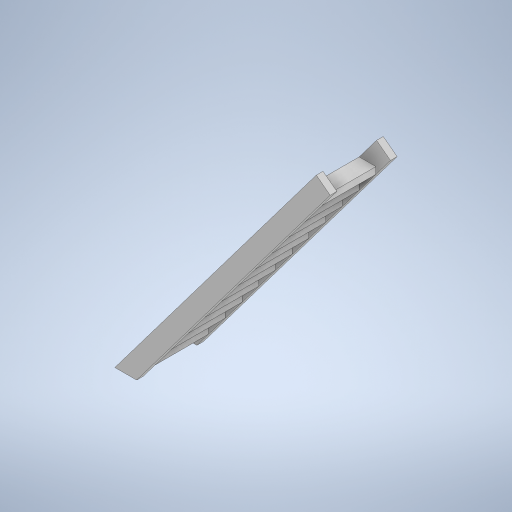
# Autodesk Inventor part: Maitri_Ladder
Saved by Autodesk Inventor 2023 (Build 270158000, 158)
## iProperties
Created: 2023-09-22
Part Number: Maitri_Ladder
Material: Generic
Document SubType Name: Modeling
Designer: maitr
Density: 1 g/cm^3
Appearance: Default
Author: maitr
Autodesk Inventor part; units mm, degrees
ref_plane "YZ Plane" through (0, 0, 0) normal (1, 0, 0) x (0, 1, 0)
ref_plane "XZ Plane" through (0, 0, 0) normal (0, 1, 0) x (-1, 0, 0)
sketch "Sketch1" plane through (0, 0, 0) normal (0, 0, 1) x (1, 0, 0)
  line L0 (0, 0) -> (3009.0751, 3993.1776)
  line L1 (0, 0) -> (5000, 0) construction
  line L2 (0, 0) -> (314.0852, 0)
  line L3 (0, 0) -> (250, 0)
  line L4 (250, 331.7612) -> (500, 331.7612)
  line L5 (500, 663.5224) -> (750, 663.5224)
  line L6 (750, 995.2836) -> (1000, 995.2836)
  line L7 (1000, 1327.0448) -> (1250, 1327.0448)
  line L8 (1250, 1658.806) -> (1500, 1658.806)
  line L9 (1500, 1990.5672) -> (1750, 1990.5672)
  line L10 (1750, 2322.3284) -> (2000, 2322.3284)
  line L11 (2000, 2654.0896) -> (2250, 2654.0896)
  line L12 (2250, 2985.8508) -> (2500, 2985.8508)
  line L13 (2500, 3317.6121) -> (2750, 3317.6121)
  line L14 (2750, 3649.3733) -> (3000, 3649.3733)
  line L15 (250, 231.7612) -> (500, 231.7612)
  line L16 (500, 563.5224) -> (750, 563.5224)
  line L17 (750, 895.2836) -> (1000, 895.2836)
  line L18 (1000, 1227.0448) -> (1250, 1227.0448)
  line L19 (1250, 1558.806) -> (1500, 1558.806)
  line L20 (1500, 1890.5672) -> (1750, 1890.5672)
  line L21 (1750, 2222.3284) -> (2000, 2222.3284)
  line L22 (2000, 2554.0896) -> (2250, 2554.0896)
  line L23 (2250, 2885.8508) -> (2500, 2885.8508)
  line L24 (2500, 3217.6121) -> (2750, 3217.6121)
  line L25 (2750, 3549.3733) -> (3000, 3549.3733)
  line L26 (500, 231.7612) -> (3000, 3549.3733)
  line L27 (3000, 3549.3733) -> (3323.7765, 3979.0392)
  line L28 (3000, 3549.3733) -> (3538, 3549.3733) construction
  line L29 (500, 231.7612) -> (314.0852, 0)
  line L30 (250, 331.7612) -> (250, 231.7612)
  line L31 (500, 331.7612) -> (500, 231.7612)
  line L32 (500, 663.5224) -> (500, 563.5224)
  line L33 (750, 663.5224) -> (750, 563.5224)
  line L34 (750, 995.2836) -> (750, 895.2836)
  line L35 (1000, 995.2836) -> (1000, 895.2836)
  line L36 (1000, 1327.0448) -> (1000, 1227.0448)
  line L37 (1250, 1327.0448) -> (1250, 1227.0448)
  line L38 (1250, 1658.806) -> (1250, 1558.806)
  line L39 (1500, 1658.806) -> (1500, 1558.806)
  line L40 (1500, 1990.5672) -> (1500, 1890.5672)
  line L41 (1750, 1990.5672) -> (1750, 1890.5672)
  line L42 (1750, 2322.3284) -> (1750, 2222.3284)
  line L43 (2000, 2322.3284) -> (2000, 2222.3284)
  line L44 (2000, 2654.0896) -> (2000, 2554.0896)
  line L45 (2250, 2654.0896) -> (2250, 2554.0896)
  line L46 (2250, 2985.8508) -> (2250, 2885.8508)
  line L47 (2500, 2985.8508) -> (2500, 2885.8508)
  line L48 (2500, 3317.6121) -> (2500, 3217.6121)
  line L49 (2750, 3317.6121) -> (2750, 3217.6121)
  line L50 (2750, 3649.3733) -> (2750, 3549.3733)
  line L51 (3000, 3649.3733) -> (3000, 3549.3733)
  line L52 (-199.9995, -0.4419) -> (2809.0756, 3992.7357)
  line L53 (-199.9995, -0.4419) -> (4800.0005, -0.4419) construction
  line L54 (500, -0.4419) -> (3509.0751, 3992.7357)
  line L55 (500, -0.4419) -> (5500, -0.4419) construction
  line L56 (-199.9995, -0.4419) -> (500, -0.4419)
  line L57 (2809.0756, 3992.7357) -> (3509.0751, 3992.7357)
  dimension "d0" = 5000
  dimension "d1" = 53
  dimension "d2" = 250
  dimension "d3" = 250
  dimension "d4" = 250
  dimension "d5" = 250
  dimension "d6" = 250
  dimension "d7" = 250
  dimension "d8" = 250
  dimension "d9" = 250
  dimension "d10" = 250
  dimension "d11" = 250
  dimension "d12" = 250
  dimension "d13" = 250
  dimension "d14" = 100
  dimension "d15" = 100
  dimension "d16" = 100
  dimension "d17" = 100
  dimension "d18" = 100
  dimension "d19" = 100
  dimension "d20" = 100
  dimension "d21" = 100
  dimension "d22" = 100
  dimension "d23" = 100
  dimension "d24" = 100
  dimension "d25" = 538
  dimension "d26" = 53
  dimension "d27" = 5000
  dimension "d28" = 53
  dimension "d29" = 200
  dimension "d30" = 5000
  dimension "d31" = 53
  constraints: 114 end point, 27 horizontal, 17 perpendicular, 3 equal length, 3 point on line, 3 vertical, 1 collinear, 14 other
  measures "d0" distance of L1.start point (3009.075, 3993.178)
  measures "d2" distance of L1.start L3.end
  measures "d3" distance of L4.start L4.end
  measures "d4" distance of L5.start L5.end
  measures "d5" distance of L6.start L6.end
  measures "d6" distance of L7.start L7.end
  measures "d7" distance of L8.start L8.end
  measures "d8" distance of L9.start L9.end
  measures "d9" distance of L10.start L10.end
  measures "d10" distance of L11.start L11.end
  measures "d11" distance of L12.start L12.end
  measures "d12" distance of L13.start L13.end
  measures "d13" distance of L14.start L14.end
  measures "d14" distance between parallel lines of L15 L4
  measures "d15" distance between parallel lines of L16 L5
  measures "d16" distance between parallel lines of L17 L6
  measures "d17" distance between parallel lines of L18 L7
  measures "d18" distance from line of L19.end L8
  measures "d19" distance between parallel lines of L20 L9
  measures "d20" distance between parallel lines of L21 L10
  measures "d21" distance between parallel lines of L22 L11
  measures "d22" distance between parallel lines of L23 L12
  measures "d23" distance between parallel lines of L24 L13
  measures "d24" distance between parallel lines of L25 L14
  measures "d25" distance of L25.end L27.end
  measures "d26" angle of L28 L27
  measures "d27" distance of L52.start L52.end
  measures "d28" angle of L53 L52
  measures "d29" distance of L1.start L52.start
  measures "d30" distance of L54.start L54.end
  measures "d31" angle of L55 L54
sketch "Sketch2" plane through (0, 0, 0) normal (1, 0, 0) x (0, 1, 0)
  point P0 (0, 0)
sketch "Sketch3" plane through (0, 0, 0) normal (0, 0, 1) x (1, 0, 0)
  point P0 (0, 0)
extrude "Extrusion1" add sketch "Sketch1" along normal blind 500 contours L4 L31 L15 L30 | L5 L33 L16 L32 | L6 L35 L17 L34 | L7 L37 L18 L36 | L8 L39 L19 L38 | L9 L41 L20 L40 | L10 L43 L21 L42 | L11 L45 L22 L44 | L12 L47 L23 L46 | L13 L49 L24 L48 | L14 L51 L25 L50
sketch "Sketch4" plane through (0, 0, 0) normal (0, 0, 1) x (1, 0, 0)
  line L0 (0, 0) -> (3009.0751, 3993.1776)
  line L1 (0, 0) -> (5000, 0) construction
  line L2 (3000, 3549.3733) -> (3000, 3649.3733) projected
  line L3 (3000, 3549.3733) -> (325.3554, 0)
  line L4 (3216.5929, 3836.8017) -> (3000, 3549.3733)
  line L5 (3216.5929, 3836.8017) -> (3009.0751, 3993.1776)
  line L6 (325.3554, 0) -> (0, 0)
  dimension "d34" = 5000
  dimension "d35" = 53
  constraints: 12 end point, 2 point on line, 1 collinear, 1 equal length, 1 horizontal, 1 perpendicular
  measures "d34" distance of L0.start L0.end
  measures "d35" angle of L1 L0
extrude "Extrusion2" add sketch "Sketch4" along normal blind 100
ref_plane "Work Plane1" through (0, 0, 500) normal (0, 0, -1) x (-1, 0, 0)
mirror "Mirror1" about plane through (0, 0, 500) normal (0, 0, -1) of "Extrusion1", "Extrusion2"
body "Solid1"
